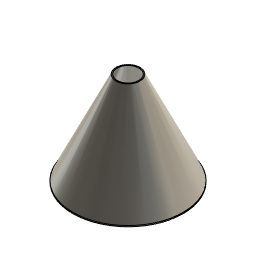
mn v2 (Autodesk Fusion 360 design; units mm, degrees)
Autodesk Fusion 360 part; units mm, degrees
sketch "スケッチ1" plane through (0, 0, 0) normal (0, 0, 1) x (1, 0, 0)
  circle A0 centre (0, 0) radius 50
  circle A1 centre (0, 0) radius 51
  dimension "d1" = 102
  constraint coincident A0.centre A1.centre
  measures "d1" diameter of A1
ref_plane "作業平面1" through (0, 0, 86) normal (0, 0, 1) x (1, 0, 0)
sketch "スケッチ2" plane through (0, 0, 86) normal (0, 0, 1) x (1, 0, 0)
  circle A0 centre (0, 0) radius 10
  circle A1 centre (0, 0) radius 11
  dimension "d3" = 20
  dimension "d4" = 22
  constraint coincident A0.centre A1.centre
  constraint concentric A0 A1
  measures "d3" diameter of A0
  measures "d4" diameter of A1
extrude "押し出し1" add sketch "スケッチ1" along normal blind 1 contours A0 | A1
sketch "スケッチ3" plane through (0, 0, 1) normal (0, 0, 1) x (-1, 0, 0)
  circle A0 centre (0, 0) radius 51
  circle A1 centre (0, 0) radius 51
  circle A2 centre (0, 0) radius 50
  dimension "d7" = 100
  constraint coincident A0.centre A1.centre
  measures "d7" diameter of A2
loft "ロフト1" add profiles "スケッチ3", "スケッチ2" section 1 section 2 contours A0 | A1
loft "ロフト2" cut profiles "スケッチ2", "スケッチ3" section 1 contours A0 section 2 contours A2
